V3D Extrusion Cable Clip v2 (Autodesk Fusion 360 design; units mm, degrees)
Autodesk Fusion 360 part; units mm, degrees
note: some values were not read from the file. Set by a fixed rule: which sketch regions a step uses.
sketch "Sketch1" plane through (0, 0, 0) normal (0, 1, 0) x (1, 0, 0)
  line L0 (15, -15) -> (-15, -15)
  line L1 (-15, -15) -> (-15, 15)
  line L2 (-15, 15) -> (15, 15)
  line L3 (15, 15) -> (15, -15)
  line L4 (15, -15) -> (-15, 15) construction
  line L5 (-15, -15) -> (15, 15) construction
  line L6 (-4.05, -15) -> (-4.05, -12.8)
  line L7 (-4.05, -12.8) -> (-11.2444, -12.8)
  line L8 (-11.2444, -12.8) -> (-4.3444, -5.9)
  line L9 (-4.3444, -5.9) -> (0, -5.9)
  line L10 (0, 0) -> (0, -15) construction
  line L11 (4.05, -15) -> (4.05, -12.8)
  line L12 (4.05, -12.8) -> (11.2444, -12.8)
  line L13 (11.2444, -12.8) -> (4.3444, -5.9)
  line L14 (4.3444, -5.9) -> (0, -5.9)
  dimension "d1" = 30
  dimension "d2" = 30
  dimension "d3" = 8.1
  dimension "d4" = 9.1
  dimension "d6" = 2.2
  dimension "d7" = 1.1
  constraint perpendicular L0 L1
  constraint parallel L0 L2
  constraint parallel L1 L3
  constraint horizontal L0
  constraint coincident L4 L10.start
  constraint coincident L5 L10.start
  constraint coincident L10.start origin
  constraint coincident L0 L6.start
  constraint perpendicular L0 L6
  constraint perpendicular L6 L7
  constraint perpendicular L6 L9
  constraint midpoint L0 L10.end
  constraint coincident L10 L9.end
  constraint symmetric L6.start L10 L11.start
  constraint symmetric L6.end L10 L11.end
  constraint symmetric L7.end L10 L12.end
  constraint symmetric L8.end L10 L13.end
  constraint symmetric L10 L9.end L14.end
  constraint perpendicular L8 L13
  measures "d1" distance of L0.start L0.end
  measures "d2" distance of L0.end L1.end
  measures "d3" distance of L6 L11
  measures "d4" distance of L0 L9
  measures "d6" distance of L0 L12
  measures "d7" distance of L4 L13
sketch "Sketch2" plane through (0, 0, 0) normal (0, 1, 0) x (1, 0, 0)
  line L0 (15, -15) -> (-15, -15) construction
  line L1 (3.5, -15) -> (3.5, -12.9)
  line L2 (3.5, -12.9) -> (8.5, -12.9)
  line L3 (8.5, -12.9) -> (4.5, -8.9)
  line L4 (3.5, -15) -> (12, -15)
  line L5 (12, -15) -> (12, -16.35)
  line L6 (12, -16.35) -> (-8.15, -16.35)
  arc A0 (-8.15, -16.35) -> (-8.15, -21.35) centre (-8.15, -18.85) ccw
  line L7 (-8.15, -21.35) -> (8, -21.35)
  line L8 (8, -21.35) -> (8, -17.75)
  line L9 (9.7071, -17.0429) -> (12, -19.3358)
  line L10 (12, -19.3358) -> (12, -22.7)
  line L11 (12, -22.7) -> (-8.15, -22.7)
  arc A1 (-8.15, -15) -> (-8.15, -22.7) centre (-8.15, -18.85) ccw
  line L12 (-8.15, -15) -> (-3.5, -15)
  line L13 (-3.5, -15) -> (-3.5, -12.9)
  line L14 (-3.5, -12.9) -> (-8.5, -12.9)
  line L15 (-11.2444, -12.8) -> (-4.3444, -5.9) construction
  line L16 (-8.5, -12.9) -> (-4.5, -8.9)
  line L17 (-4.5, -8.9) -> (4.5, -8.9)
  line L18 (-12, -18.85) -> (-12, -26.3495) construction
  line L19 (-15, -15) -> (-15, 15)
  line L20 (15, 15) -> (15, -15)
  line L21 (0, 0) -> (0, -24.1039) construction
  arc A2 (9.7071, -17.0429) -> (8, -17.75) centre (9, -17.75) ccw
  point P0 (8, -15.3358)
  dimension "d8" = 3
  dimension "d9" = 3
  dimension "d12" = 1.35
  dimension "d13" = 4
  dimension "d14" = 7
  dimension "d15" = 17
  dimension "d18" = 4
  dimension "d19" = 5
  dimension "d20" = 45
  dimension "d25" = 1
  dimension "d26" = 1.4
  dimension "d40" = 2.1
  constraint perpendicular L0 L1
  constraint perpendicular L1 L2
  constraint perpendicular L1 L4
  constraint perpendicular L4 L5
  constraint perpendicular L5 L6
  constraint tangent L6 A0
  constraint tangent A0 L7
  constraint horizontal L7
  constraint perpendicular L7 L8
  constraint vertical L10
  constraint perpendicular L10 L11
  constraint tangent L11 A1
  constraint tangent A1 L12
  constraint horizontal L12
  constraint concentric A0 A1
  constraint perpendicular L12 L13
  constraint perpendicular L13 L14
  constraint parallel L15 L16
  constraint horizontal L17
  constraint midpoint A1 L18.start
  constraint tangent A1 L18
  constraint vertical L18
  constraint collinear L4 L12
  constraint collinear L2 L14
  constraint equal L2 L14
  constraint collinear L5 L10
  constraint coincident L21.start origin
  constraint perpendicular L11 L21
  constraint symmetric L1 L13 L21
  constraint perpendicular L3 L16
  constraint coincident P0 L9
  constraint coincident P0 L8
  constraint tangent L9 A2
  constraint tangent L8 A2
  constraint collinear L0 L4
  measures "d8" distance of L18 L19
  measures "d9" distance of L5 L20
  measures "d12" distance of L4.end L5.end
  measures "d13" distance of L2 L17
  measures "d14" distance of L1 L13
  measures "d15" distance of L2.end L14.end
  measures "d18" distance of L8 L10
  measures "d19" distance of L6 L7
  measures "d20" angle of L6 L9
  measures "d25" radius of A2
  measures "d26" distance of L6 A2.centre
  measures "d40" distance of L2 L4
extrude "Extrude1" add sketch "Sketch2" along normal mid plane 7
chamfer "Chamfer1" distance 2 angle 45 4 edges at (-3.5, -3.5, 13.95) (3.5, -3.5, 13.95) (3.5, 3.5, 13.95) (-3.5, 3.5, 13.95)
sketch "Sketch3" plane through (0, 0, 0) normal (0, 0, 1) x (1, 0, 0)
  circle A0 centre (0, 0) radius 4
  circle A1 centre (0, 0) radius 8.25
  dimension "d24" = 8
  dimension "d29" = 16.5
  constraint coincident A0.centre A1.centre
  constraint concentric A0 A1
  measures "d24" diameter of A0
  measures "d29" diameter of A1
fillet "Fillet1" radius 2.5 2 edges at (8, 0, 21.35) (12, 0, 22.7)
fillet "Fillet2" radius 1 4 edges at (8.5, 0, 12.9) (4.5, 0, 8.9) (-4.5, 0, 8.9) (-8.5, 0, 12.9)
sketch "Sketch4" plane through (0, 0, 0) normal (0, 1, 0) x (1, 0, 0)
  line L0 (-1.5, -15) -> (-8.15, -15)
  line L1 (-6.325, -15) -> (-6.325, -14.9)
  arc A0 (-4.825, -15) -> (-6.325, -14.9) centre (-6.325, -26.2) ccw
  line L2 (-6.325, -14.9) -> (-5.7947, -14.9) construction
  dimension "d30" = 0.1
  dimension "d31" = 1.5
  constraint coincident L0 L1.start
  constraint perpendicular L0 L1
  constraint midpoint L0 A0.start
  constraint tangent A0 L2
  constraint perpendicular L1 L2
  measures "d30" distance of L0 L1.end
  measures "d31" distance of L1 A0.start
equation "d12 = ( 0.45 * 3 ) * 1 mm"
